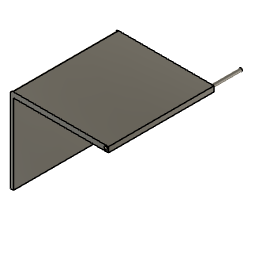
왼쪽 범퍼 문 (Autodesk Fusion 360 design; units mm, degrees)
Autodesk Fusion 360 part; units mm, degrees
sketch "스케치1" plane through (0, 0, 0) normal (0, 1, 0) x (1, 0, 0)
  line L0 (0, 0) -> (6, 0)
  line L1 (0, 0) -> (0, -62)
  line L2 (0, -62) -> (93, -62)
  line L3 (6, 0) -> (6, -57)
  line L4 (6, -57) -> (93, -57)
  line L5 (93, -57) -> (93, -62)
  line L6 (6, -57) -> (3, -57)
  line L7 (3, -57) -> (3, 0)
  line L8 (3, 0) -> (6, 0)
  line L9 (6, 0) -> (6, -57)
  dimension "d1" = 6
  dimension "d2" = 62
  dimension "d3" = 93
  dimension "d4" = 57
  constraint coincident L0.start L1.start
  constraint horizontal L0
  constraint perpendicular L0 L1
  constraint perpendicular L1 L2
  constraint perpendicular L0 L3
  constraint perpendicular L3 L4
  constraint perpendicular L2 L5
  constraint horizontal L6
  constraint vertical L7
  constraint horizontal L8
  constraint vertical L9
  constraint midpoint L0 L7.end
  measures "d1" distance of L0.start L0.end
  measures "d2" distance of L0.start L1.end
  measures "d3" distance of L1.end L2.end
  measures "d4" distance of L0.end L3.end
extrude "돌출1" add sketch "스케치1" along normal blind 100 contours L0 L1 L2 L4 L5 L6 L7
sketch "스케치2" plane through (0, 0, 0) normal (0, -1, 0) x (1, 0, 0)
  line L0 (0, 62) -> (0, 0)
  line L1 (0, 0) -> (3, 0)
  line L2 (3, 57) -> (93, 57)
  line L3 (93, 57) -> (93, 62)
  line L4 (93, 62) -> (0, 62)
  line L5 (93, 62) -> (88, 62)
  line L6 (88, 62) -> (88, 57)
  line L7 (88, 57) -> (93, 57)
  line L8 (93, 57) -> (93, 62)
  circle A0 centre (90.5, 59.5) radius 1.6
  line L9 (3, 0) -> (3, 57)
  dimension "d7" = 3.2
  constraint horizontal L5
  constraint vertical L6
  constraint horizontal L7
  constraint vertical L8
  constraint coincident L2 L6.end
  constraint coincident L3.end L4.start
  measures "d7" diameter of A0
extrude "돌출2" cut sketch "스케치2" against normal blind 35 contours A0
sketch "스케치3" plane through (0, 100, 0) normal (0, 1, 0) x (-1, 0, 0)
  line L0 (0, 0) -> (0, 62)
  line L1 (0, 62) -> (-93, 62)
  line L2 (-93, 62) -> (-93, 57)
  line L3 (-93, 57) -> (-3, 57)
  line L4 (-3, 0) -> (0, 0)
  line L5 (-93, 62) -> (-87, 62)
  line L6 (-87, 62) -> (-87, 57)
  line L7 (-87, 57) -> (-93, 57)
  line L8 (-93, 57) -> (-93, 62)
  circle A0 centre (-90, 59.5) radius 1.5
  line L9 (-3, 57) -> (-3, 0)
  dimension "d10" = 3
  constraint horizontal L5
  constraint vertical L6
  constraint horizontal L7
  constraint vertical L8
  constraint coincident L1.end L2.start
  measures "d10" diameter of A0
extrude "돌출3" add sketch "스케치3" along normal blind 30 contours A0
fillet "필렛1" radius 1.5 1 edges at (91.3985, 130, 58.9576)
fillet "필렛2" radius 2.5 1 edges at (0, 50, 62)
extrude "돌출4" add 1 faces at (1, 66.6667, 0) along direction (0, 0, -1) blind 18.755
